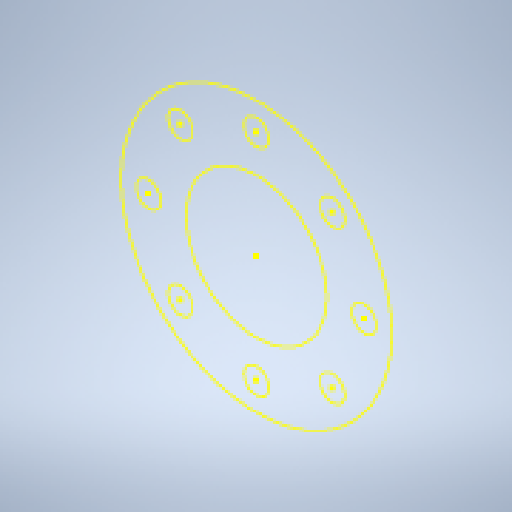
# Autodesk Inventor part: _thigh_adt_body
Saved by Autodesk Inventor 2024.3 (Build 283343000, 343)
## iProperties
Created: 2024-09-06
Part Number: _thigh_adt_body
Material: 일반
Document SubType Name: Modeling
Designer: gretc
Density: 1 g/cm^3
Appearance: 기본값
Author: gretc
Autodesk Inventor part; units mm, degrees
ref_plane "YZ Plane" through (0, 0, 0) normal (1, 0, 0) x (0, 1, 0)
ref_plane "XZ Plane" through (0, 0, 0) normal (0, 1, 0) x (-1, 0, 0)
ref_plane "XY Plane" through (0, 0, 0) normal (0, 0, 1) x (1, 0, 0)
sketch "스케치1" plane through (0, 0, 0) normal (0, 0, 1) x (1, 0, 0)
  circle A0 centre (0, 0) radius 13.8 projected
  circle A1 centre (0, 0) radius 7.2 projected
  circle A2 centre (0, -11) radius 1.2813 projected
  circle A3 centre (-7.7782, -7.7782) radius 1.2813 projected
  circle A4 centre (-11, 0) radius 1.2813 projected
  circle A5 centre (-7.7782, 7.7782) radius 1.2813 projected
  circle A6 centre (0, 11) radius 1.2813 projected
  circle A7 centre (7.7782, 7.7782) radius 1.2813 projected
  circle A8 centre (11, 0) radius 1.2813 projected
  circle A9 centre (7.7782, -7.7782) radius 1.2813 projected
  circle A10 centre (0, 0) radius 3.15 projected
  circle A11 centre (0, 0) radius 3.5972
  line L0 (0, -3.5972) -> (0, 3.5972)
  line L1 (0, 3.5972) -> (17.7956, 3.5972)
  line L2 (17.7956, 3.5972) -> (17.7956, -3.5972)
  line L3 (17.7956, -3.5972) -> (0, -3.5972)
  line L4 (-54.4347, 13.8) -> (-54.4347, -13.8) projected
  line L5 (0, -13.8) -> (0, 13.8)
  line L6 (0, 13.8) -> (-54.4347, 13.8)
  line L7 (-54.4347, 13.8) -> (-54.4347, -13.8)
  line L8 (-54.4347, -13.8) -> (0, -13.8)
  point P0 (0, 0)
  point P1 (6.237, 3.5972)
  point P2 (13.3229, 3.5972)
  point P3 (13.3229, -3.5972)
  point P4 (6.237, -3.5972)
  constraints: 16 end point, 4 parallel, 4 point on circle, 2 perpendicular, 2 vertical, 1 centre point, 1 coincident
extrude "돌출1" add sketch "스케치1" along normal blind 6 contours L5 A6 A1 A2 A0 | A0 L1 A1 L5 A6 | A0 L8 L4 L6 | L5 A2 A1 L3 A0
sketch "스케치2" plane through (-54.4347, -13.8, 0) normal (-1, 0, 0) x (0, 0, 1)
  line L0 (0, 13.8) -> (6, 13.8)
  line L1 (6, 15.0812) -> (6, 12.5187) projected
  line L2 (0, 13.8) -> (3, 13.8)
  line L3 (3, 13.8) -> (3, 0)
  line L4 (0, 0) -> (6, 0) projected
  line L5 (3, 0) -> (3, 9.2)
  line L6 (3, 9.2) -> (3, 18.4)
  circle A0 centre (3, 18.4) radius 1.35
  circle A1 centre (3, 9.2) radius 1.35
  dimension "d2" = 3
  dimension "d3" = 9.2
  dimension "d4" = 9.2
  dimension "d5" = 2.7
  dimension "d6" = 2.7
  constraints: 10 end point, 3 midpoint, 2 centre point, 2 coincident, 2 point on line
  measures "d2" distance of L0.start L2.end
  measures "d3" distance of L3.end L5.end
  measures "d4" distance of L5.end L6.end
  measures "d5" diameter of A0
  measures "d6" diameter of A1
extrude "돌출2" cut sketch "스케치2" against normal blind 3
sketch "스케치3" plane through (0, 0, 6) normal (0, 0, 1) x (1, 0, 0)
  line L0 (-50.4347, -2.45) -> (-50.4347, -6.45) projected
  line L1 (-50.4347, 7.3745) -> (-50.4347, 3.3745) projected
  line L2 (-54.4347, 13.8) -> (-54.4347, -13.8) projected
  line L3 (-54.4347, 5.2526) -> (-50.4347, 5.2526)
  line L4 (-54.4347, -4.5845) -> (-50.4347, -4.5845)
  line L5 (-51.4347, -2.5845) -> (-51.4347, -6.5845)
  line L6 (-51.4347, -6.5845) -> (-49.4347, -6.5845)
  line L7 (-49.4347, -6.5845) -> (-49.4347, -2.5845)
  line L8 (-49.4347, -2.5845) -> (-51.4347, -2.5845)
  line L9 (-51.4347, -2.5845) -> (-49.4347, -6.5845) construction
  line L10 (-51.4347, -6.5845) -> (-49.4347, -2.5845) construction
  line L11 (-51.4347, 7.2526) -> (-51.4347, 3.2526)
  line L12 (-51.4347, 3.2526) -> (-49.4347, 3.2526)
  line L13 (-49.4347, 3.2526) -> (-49.4347, 7.2526)
  line L14 (-49.4347, 7.2526) -> (-51.4347, 7.2526)
  line L15 (-51.4347, 7.2526) -> (-49.4347, 3.2526) construction
  line L16 (-51.4347, 3.2526) -> (-49.4347, 7.2526) construction
  point P0 (0, 0)
  dimension "d9" = 4
  dimension "d10" = 2
  dimension "d11" = 4
  dimension "d12" = 2
  constraints: 28 end point, 4 midpoint, 4 parallel, 4 perpendicular, 4 point on line, 2 vertical
  measures "d9" distance of L5.start L5.end
  measures "d10" distance of L6.end L5.end
  measures "d11" distance of L11.start L11.end
  measures "d12" distance between parallel lines of L11 L13
extrude "돌출3" cut sketch "스케치3" against normal blind 4
